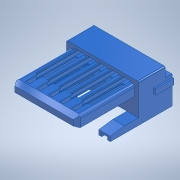
# Autodesk Inventor part: USB 3.0 A Recepticle Insert Fit
Saved by Autodesk Inventor 2020.1 (Build 241239000, 239)
## iProperties
Created: 2019-11-21
Part Number: USB 3.0 A Recepticle Insert Fit
Material: PBT Plastic
Document SubType Name: Modeling
Designer: S. Lee
Mass: 0.400509 g
Surface Area: 10.671 cm^2
Volume: 0.305732 cm^3
Density: 1.31 g/cm^3
Appearance: PBT Blue Pantone 300C
Author: S. Lee
Autodesk Inventor part; units mm, degrees
(part 1 of 2)
ref_plane "YZ Plane" through (0, 0, 0) normal (1, 0, 0) x (0, 1, 0)
ref_plane "XZ Plane" through (0, 0, 0) normal (0, 1, 0) x (-1, 0, 0)
sketch "Sketch1" plane through (0, 0, 0) normal (0, 1, 0) x (-1, 0, 0)
  line L0 (6.55, -2.62) -> (6.55, -5.82)
  line L1 (-6.55, -5.82) -> (-6.55, -2.62)
  line L2 (6.25, -2.62) -> (6.25, 0)
  line L3 (-6.25, 0) -> (-6.25, -2.62)
  line L4 (5.55, 0) -> (5.55, 9.284)
  line L5 (5.05, 10.15) -> (-5.05, 10.15)
  line L6 (-5.55, 9.284) -> (-5.55, 0)
  line L7 (6.25, 0) -> (5.55, 0)
  line L8 (-5.55, 0) -> (-6.25, 0)
  line L9 (-6.55, -2.62) -> (-6.25, -2.62)
  line L10 (6.25, -2.62) -> (6.55, -2.62)
  line L11 (4.605, 9.55) -> (3.395, 9.55)
  line L12 (3.395, 9.55) -> (3.395, 8)
  line L13 (3.395, 8) -> (4.605, 8)
  line L14 (4.605, 8) -> (4.605, 9.55)
  line L15 (2.605, 9.55) -> (1.395, 9.55)
  line L16 (1.395, 9.55) -> (1.395, 8)
  line L17 (1.395, 8) -> (2.605, 8)
  line L18 (2.605, 8) -> (2.605, 9.55)
  line L19 (0.605, 9.55) -> (-0.605, 9.55)
  line L20 (-0.605, 9.55) -> (-0.605, 8)
  line L21 (-0.605, 8) -> (0.605, 8)
  line L22 (0.605, 8) -> (0.605, 9.55)
  line L23 (-1.395, 9.55) -> (-2.605, 9.55)
  line L24 (-2.605, 9.55) -> (-2.605, 8)
  line L25 (-2.605, 8) -> (-1.395, 8)
  line L26 (-1.395, 8) -> (-1.395, 9.55)
  line L27 (-3.395, 9.55) -> (-4.605, 9.55)
  line L28 (-4.605, 9.55) -> (-4.605, 8)
  line L29 (-4.605, 8) -> (-3.395, 8)
  line L30 (-3.395, 8) -> (-3.395, 9.55)
  line L31 (4.05, 6.4) -> (2.95, 6.4)
  line L32 (2.95, 6.4) -> (2.95, -2.82)
  line L33 (4.05, -2.82) -> (4.05, 6.4)
  line L34 (1.55, 6.4) -> (0.45, 6.4)
  line L35 (0.45, 6.4) -> (0.45, -2.82)
  line L36 (1.55, -2.82) -> (1.55, 6.4)
  line L37 (-0.45, 6.4) -> (-1.55, 6.4)
  line L38 (-1.55, 6.4) -> (-1.55, -2.82)
  line L39 (-0.45, -2.82) -> (-0.45, 6.4)
  line L40 (-2.95, 6.4) -> (-4.05, 6.4)
  line L41 (-4.05, 6.4) -> (-4.05, -2.82)
  line L42 (-2.95, -2.82) -> (-2.95, 6.4)
  line L43 (-5.2, -5.82) -> (-5.2, -2.82)
  line L44 (5.2, -2.82) -> (5.2, -5.82)
  line L45 (-5.2, -2.82) -> (-4.05, -2.82)
  line L46 (-2.95, -2.82) -> (-1.55, -2.82)
  line L47 (-0.45, -2.82) -> (0.45, -2.82)
  line L48 (1.55, -2.82) -> (2.95, -2.82)
  line L49 (4.05, -2.82) -> (5.2, -2.82)
  line L50 (6.55, -5.82) -> (5.2, -5.82)
  line L51 (-5.2, -5.82) -> (-6.55, -5.82)
  line L52 (0, -9.014) -> (0, 13.344) projected
  line L53 (4.05, -2.82) -> (2.95, -2.82) construction
  line L54 (1.55, -2.82) -> (0.45, -2.82) construction
  line L55 (-0.45, -2.82) -> (-1.55, -2.82) construction
  line L56 (-2.95, -2.82) -> (-4.05, -2.82) construction
  line L57 (-3.5, 6.4) -> (-3.5, -2.82) construction
  line L58 (-1, 6.4) -> (-1, -2.82) construction
  line L59 (1, 6.4) -> (1, -2.82) construction
  line L60 (3.5, 6.4) -> (3.5, -2.82) construction
  line L61 (5.05, 10.15) -> (5.55, 9.284)
  line L62 (-5.05, 10.15) -> (-5.55, 9.284)
  line L63 (4, 9.55) -> (4, 8) construction
  line L64 (4.605, 8.775) -> (3.395, 8.775) construction
  line L65 (2.605, 8.775) -> (1.395, 8.775) construction
  line L66 (2, 9.55) -> (2, 8) construction
  line L67 (0, 9.55) -> (0, 8) construction
  line L68 (0.605, 8.775) -> (-0.605, 8.775) construction
  line L69 (-1.395, 8.775) -> (-2.605, 8.775) construction
  line L70 (-2, 9.55) -> (-2, 8) construction
  line L71 (-4, 9.55) -> (-4, 8) construction
  line L72 (-3.395, 8.775) -> (-4.605, 8.775) construction
  line L73 (9.17, 0) -> (-9.17, 0) construction
  line L74 (5.55, 5.65) -> (-5.55, 5.65) construction
  point P0 (0, 0)
  point P1 (5.55, 10.15)
  point P2 (-5.55, 10.15)
  dimension "d0" = 10.4
  dimension "d2" = 13.1
  dimension "d3" = 12.5
  dimension "d4" = 11.1
  dimension "d5" = 3.2
  dimension "d6" = 3
  dimension "d7" = 1.1
  dimension "d8" = 1
  dimension "d9" = 1
  dimension "d10" = 3.5
  dimension "d11" = 3.5
  dimension "d12" = 2.15
  dimension "d14" = 1.21
  dimension "d15" = 10.15
  dimension "d16" = 15.97
  dimension "d17" = 0.5
  dimension "d18" = 60
  dimension "d19" = 0.5
  dimension "d20" = 60
  dimension "d21" = 2
  dimension "d22" = 4
  dimension "d23" = 2
  dimension "d24" = 4
  dimension "d25" = 0.6
  dimension "d27" = 4.5
  dimension "d28" = 0.75
  constraints: 146 end point, 30 collinear, 28 midpoint, 22 parallel, 12 horizontal, 12 perpendicular, 6 point on line, 4 other
  measures "d0" distance between parallel lines of L43 L44
  measures "d2" distance between parallel lines of L1 L0
  measures "d3" distance between parallel lines of L3 L2
  measures "d4" distance between parallel lines of L6 L4
  measures "d5" distance of L0.start L0.end
  measures "d6" distance of L44.start L44.end
  measures "d7" distance of L40.start L40.end
  measures "d8" distance between parallel lines of L58 L52
  measures "d9" distance between parallel lines of L52 L59
  measures "d10" distance between parallel lines of L52 L60
  measures "d11" distance between parallel lines of L52 L57
  measures "d12" distance between parallel lines of L5 L29
  measures "d14" distance between parallel lines of L30 L28
  measures "d15" distance of L4.start point (5.55, 10.15)
  measures "d16" distance between parallel lines of L51 L5
  measures "d17" distance of L5.start point (5.55, 10.15)
  measures "d18" angle of L5 L61
  measures "d19" distance of L5.end point (-5.55, 10.15)
  measures "d20" angle of L5 L62
  measures "d21" distance between parallel lines of L66 L52
  measures "d22" distance between parallel lines of L63 L52
  measures "d23" distance between parallel lines of L70 L52
  measures "d24" distance between parallel lines of L71 L52
  measures "d25" distance between parallel lines of L27 L5
  measures "d27" distance between parallel lines of L74 L5
  measures "d28" distance between parallel lines of L74 L40
extrude "Extrusion1" add sketch "Sketch1" along normal blind 0.32 contours L0 L50 L44 L49 L33 L31 L32 L48 L36 L34 L35 L47 L52 L21 L22 L19 L5 L61 L4 L7 L2 L10 | L52 L19 L20 L21 L47 L39 L37 L38 L46 L42 L40 L41 L45 L43 L51 L1 L9 L3 L8 L6 L62 L5
sketch "Sketch2" plane through (0, 0.32, 0) normal (0, 1, 0) x (1, 0, 0)
  line L0 (-4.75, -7.72) -> (4.75, -7.72)
  line L1 (5.55, -9.284) -> (5.55, 0) projected
  line L2 (-5.55, 0) -> (-5.55, -9.284) projected
  line L3 (5.55, -9.284) -> (5.55, 0) projected
  line L4 (5.55, -9.284) -> (5.55, 0)
  line L5 (6.25, 0) -> (6.25, 2.62) projected
  line L6 (6.25, 0) -> (5.55, 0)
  line L7 (6.25, 0) -> (6.25, 5.82)
  line L8 (6.55, 5.82) -> (5.2, 5.82) projected
  line L9 (5.05, -10.15) -> (5.55, -9.284) projected
  line L10 (5.55, -9.284) -> (5.05, -10.15)
  line L11 (5.05, -10.15) -> (-5.05, -10.15)
  line L12 (-5.55, -9.284) -> (-5.05, -10.15) projected
  line L13 (-5.05, -10.15) -> (-5.55, -9.284)
  line L14 (-6.25, 0) -> (-5.55, 0) projected
  line L15 (-5.55, -9.284) -> (-5.55, 0)
  line L16 (-5.55, 0) -> (-6.25, 0)
  line L17 (-6.25, 0) -> (-6.25, 5.82)
  line L18 (-5.2, 5.82) -> (-6.55, 5.82) projected
  line L19 (-5.2, 2.82) -> (-5.2, 5.82) projected
  line L20 (-5.2, 2.82) -> (-5.2, 5.82)
  line L21 (4.75, 2.82) -> (5.2, 2.82)
  line L22 (5.2, 2.82) -> (5.2, 5.82)
  line L23 (-6.25, 5.82) -> (-5.2, 5.82)
  line L24 (5.2, 5.82) -> (6.25, 5.82)
  line L25 (4.75, -7.72) -> (4.75, 2.82)
  line L26 (5.2, 5.82) -> (5.2, 2.82) projected
  line L27 (-4.05, 2.82) -> (-5.2, 2.82) projected
  line L28 (-5.2, 2.82) -> (-4.75, 2.82)
  line L29 (-4.05, 2.82) -> (-5.2, 2.82) projected
  line L30 (-4.75, 2.82) -> (-4.75, -7.72)
  line L31 (5.2, 2.82) -> (4.05, 2.82) projected
  line L32 (-4.605, -8) -> (-3.395, -8) projected
  line L33 (-3.395, -9.55) -> (-4.605, -9.55) projected
  line L34 (-4.605, -9.55) -> (-3.395, -9.55)
  line L35 (-3.395, -9.55) -> (-3.395, -8)
  line L36 (-3.395, -8) -> (-4.605, -8)
  line L37 (-4.605, -8) -> (-4.605, -9.55)
  line L38 (-1.395, -9.55) -> (-2.605, -9.55) projected
  line L39 (-2.605, -8) -> (-1.395, -8) projected
  line L40 (-2.605, -9.55) -> (-1.395, -9.55)
  line L41 (-1.395, -9.55) -> (-1.395, -8)
  line L42 (-1.395, -8) -> (-2.605, -8)
  line L43 (-2.605, -8) -> (-2.605, -9.55)
  line L44 (0.605, -9.55) -> (-0.605, -9.55) projected
  line L45 (0.605, -8) -> (0.605, -9.55) projected
  line L46 (-0.605, -9.55) -> (0.605, -9.55)
  line L47 (0.605, -9.55) -> (0.605, -8)
  line L48 (0.605, -8) -> (-0.605, -8)
  line L49 (-0.605, -8) -> (-0.605, -9.55)
  line L50 (1.395, -9.55) -> (1.395, -8) projected
  line L51 (1.395, -9.55) -> (2.605, -9.55)
  line L52 (2.605, -9.55) -> (2.605, -8)
  line L53 (2.605, -8) -> (1.395, -8)
  line L54 (1.395, -8) -> (1.395, -9.55)
  line L55 (3.395, -9.55) -> (3.395, -8) projected
  line L56 (3.395, -8) -> (4.605, -8) projected
  line L57 (3.395, -9.55) -> (4.605, -9.55)
  line L58 (4.605, -9.55) -> (4.605, -8)
  line L59 (4.605, -8) -> (3.395, -8)
  line L60 (3.395, -8) -> (3.395, -9.55)
  point P0 (0, 0)
  dimension "d34" = 0.8
  dimension "d35" = 0.8
  dimension "d36" = 0.28
  constraints: 76 end point, 12 parallel, 10 perpendicular, 9 horizontal, 8 collinear, 4 point on line, 1 vertical
  measures "d34" distance between parallel lines of L2 L30
  measures "d35" distance between parallel lines of L1 L25
  measures "d36" distance between parallel lines of L0 L32
extrude "Extrusion2" add sketch "Sketch2" along normal blind 0.5
sketch "Sketch3" plane through (0, 0.82, 0) normal (0, 1, 0) x (1, 0, 0)
  line L0 (6.25, 5.82) -> (6.25, 2.62) projected
  line L1 (6.25, 0) -> (6.25, 4.62)
  line L2 (6.25, 4.62) -> (-6.25, 4.62)
  line L3 (-6.25, 4.62) -> (-6.25, 0)
  line L4 (-5.2, 5.82) -> (-6.25, 5.82) projected
  line L5 (-5.55, 0) -> (-5.55, -9.284) projected
  line L6 (-5.55, 0) -> (-5.55, -9.284)
  line L7 (-5.55, -9.284) -> (-5.05, -10.15) projected
  line L8 (-5.55, -9.284) -> (-5.05, -10.15)
  line L9 (5.05, -10.15) -> (5.55, -9.284) projected
  line L10 (-5.05, -10.15) -> (5.05, -10.15)
  line L11 (5.05, -10.15) -> (5.55, -9.284)
  line L12 (5.55, -9.284) -> (5.55, 0) projected
  line L13 (5.55, -9.284) -> (5.55, 0)
  line L14 (-6.25, 0) -> (-5.55, 0)
  line L15 (5.55, 0) -> (6.25, 0)
  line L16 (-5.55, 0) -> (-4.05, 0)
  line L17 (4.05, 0) -> (5.55, 0)
  line L18 (-3.395, -9.55) -> (-4.605, -9.55) projected
  line L19 (-3.395, -8) -> (-3.395, -9.55) projected
  line L20 (-4.605, -9.55) -> (-3.395, -9.55)
  line L21 (-3.395, -9.55) -> (-3.395, -8)
  line L22 (-3.395, -8) -> (-4.605, -8)
  line L23 (-4.605, -8) -> (-4.605, -9.55)
  line L24 (-1.395, -9.55) -> (-2.605, -9.55) projected
  line L25 (-2.605, -8) -> (-1.395, -8) projected
  line L26 (-2.605, -9.55) -> (-1.395, -9.55)
  line L27 (-1.395, -9.55) -> (-1.395, -8)
  line L28 (-1.395, -8) -> (-2.605, -8)
  line L29 (-2.605, -8) -> (-2.605, -9.55)
  line L30 (0.605, -8) -> (0.605, -9.55) projected
  line L31 (-0.605, -9.55) -> (0.605, -9.55)
  line L32 (0.605, -9.55) -> (0.605, -8)
  line L33 (0.605, -8) -> (-0.605, -8)
  line L34 (-0.605, -8) -> (-0.605, -9.55)
  line L35 (2.605, -9.55) -> (1.395, -9.55) projected
  line L36 (1.395, -9.55) -> (2.605, -9.55)
  line L37 (2.605, -9.55) -> (2.605, -8)
  line L38 (2.605, -8) -> (1.395, -8)
  line L39 (1.395, -8) -> (1.395, -9.55)
  line L40 (4.605, -9.55) -> (3.395, -9.55) projected
  line L41 (3.395, -8) -> (4.605, -8) projected
  line L42 (3.395, -9.55) -> (4.605, -9.55)
  line L43 (4.605, -9.55) -> (4.605, -8)
  line L44 (4.605, -8) -> (3.395, -8)
  line L45 (3.395, -8) -> (3.395, -9.55)
  line L46 (5.55, 0) -> (6.25, 0) projected
  line L47 (-6.25, 4.62) -> (6.25, 4.62)
  line L48 (6.25, 4.62) -> (6.25, 0)
  line L49 (6.25, 0) -> (-6.25, 0)
  line L50 (-6.25, 0) -> (-6.25, 4.62)
  line L51 (-4.605, -7.4) -> (-3.395, -7.4)
  line L52 (-3.395, -7.4) -> (-3.395, 0)
  line L53 (-3.395, 0) -> (-4.605, 0)
  line L54 (-4.605, 0) -> (-4.605, -7.4)
  line L55 (-2.605, -7.4) -> (-1.395, -7.4)
  line L56 (-1.395, -7.4) -> (-1.395, 0)
  line L57 (-1.395, 0) -> (-2.605, 0)
  line L58 (-2.605, 0) -> (-2.605, -7.4)
  line L59 (-0.605, -7.4) -> (0.605, -7.4)
  line L60 (0.605, -7.4) -> (0.605, 0)
  line L61 (0.605, 0) -> (-0.605, 0)
  line L62 (-0.605, 0) -> (-0.605, -7.4)
  line L63 (1.395, -7.4) -> (2.605, -7.4)
  line L64 (2.605, -7.4) -> (2.605, 0)
  line L65 (2.605, 0) -> (1.395, 0)
  line L66 (1.395, 0) -> (1.395, -7.4)
  line L67 (3.395, 0) -> (4.605, 0)
  line L68 (4.605, 0) -> (4.605, -7.4)
  line L69 (4.605, -7.4) -> (3.395, -7.4)
  line L70 (3.395, -7.4) -> (3.395, 0)
  line L71 (-4.605, -9.55) -> (-4.605, -8) projected
  line L72 (-3.395, -8) -> (-3.395, -9.55) projected
  line L73 (-2.605, -9.55) -> (-2.605, -8) projected
  line L74 (-1.395, -8) -> (-1.395, -9.55) projected
  line L75 (-0.605, -9.55) -> (-0.605, -8) projected
  line L76 (0.605, -8) -> (0.605, -9.55) projected
  line L77 (1.395, -9.55) -> (1.395, -8) projected
  line L78 (2.605, -8) -> (2.605, -9.55) projected
  line L79 (3.395, -9.55) -> (3.395, -8) projected
  line L80 (4.605, -8) -> (4.605, -9.55) projected
  point P0 (-0.605, 0)
  dimension "d39" = 1.2
  dimension "d88" = 0.6
  constraints: 112 end point, 25 parallel, 17 collinear, 14 perpendicular, 10 horizontal, 6 point on line, 1 vertical
  measures "d39" distance between parallel lines of L2 L4
  measures "d88" distance between parallel lines of L51 L22
extrude "Extrusion3" add sketch "Sketch3" along normal blind 0.02 contours L0 L1 L15 L17 L49 L16 L14 L3 L2 | L12 L9 L10 L7 L5 L16 L54 L51 L52 L49 L58 L55 L56 L62 L59 L60 L66 L63 L64 L70 L69 L68 L17
sketch "Sketch5" plane through (0, 0.84, 0) normal (0, 1, 0) x (1, 0, 0)
  line L0 (-6.25, 0) -> (-5.55, 0) projected
  line L1 (5.2, 4.62) -> (6.25, 4.62) projected
  line L2 (-6.25, 0) -> (6.25, 0)
  line L3 (6.25, 0) -> (6.25, 4.62)
  line L4 (6.25, 4.62) -> (-6.25, 4.62)
  line L5 (-6.25, 4.62) -> (-6.25, 0)
  line L6 (-4.605, 0) -> (-3.395, 0) projected
  line L7 (-3.395, -8) -> (-3.395, -9.55) projected
  line L8 (-4.605, 0) -> (-3.395, 0)
  line L9 (-3.395, 0) -> (-3.395, -9.05)
  line L10 (-3.395, -9.05) -> (-4.605, -9.05)
  line L11 (-4.605, -9.05) -> (-4.605, 0)
  line L12 (-2.605, -7.4) -> (-2.605, 0) projected
  line L13 (-1.395, -8) -> (-1.395, -9.55) projected
  line L14 (-2.605, 0) -> (-1.395, 0)
  line L15 (-1.395, 0) -> (-1.395, -9.05)
  line L16 (-1.395, -9.05) -> (-2.605, -9.05)
  line L17 (-2.605, -9.05) -> (-2.605, 0)
  line L18 (-0.605, 0) -> (0.605, 0) projected
  line L19 (0.605, -8) -> (0.605, -9.55) projected
  line L20 (-0.605, 0) -> (0.605, 0)
  line L21 (0.605, 0) -> (0.605, -9.05)
  line L22 (0.605, -9.05) -> (-0.605, -9.05)
  line L23 (-0.605, -9.05) -> (-0.605, 0)
  line L24 (1.395, 0) -> (2.605, 0) projected
  line L25 (2.605, -8) -> (2.605, -9.55) projected
  line L26 (1.395, 0) -> (2.605, 0)
  line L27 (2.605, 0) -> (2.605, -9.05)
  line L28 (2.605, -9.05) -> (1.395, -9.05)
  line L29 (1.395, -9.05) -> (1.395, 0)
  line L30 (3.395, 0) -> (4.605, 0) projected
  line L31 (4.605, -8) -> (4.605, -9.55) projected
  line L32 (3.395, 0) -> (4.605, 0)
  line L33 (4.605, 0) -> (4.605, -9.05)
  line L34 (4.605, -9.05) -> (3.395, -9.05)
  line L35 (3.395, -9.05) -> (3.395, 0)
  line L36 (-3.395, -9.55) -> (-4.605, -9.55) projected
  line L37 (-5.55, 0) -> (-5.55, -9.284) projected
  line L38 (-5.55, 0) -> (-5.55, -9.284)
  line L39 (-5.55, -9.284) -> (-5.05, -10.15)
  line L40 (-5.05, -10.15) -> (5.05, -10.15) projected
  line L41 (-5.05, -10.15) -> (5.05, -10.15)
  line L42 (5.05, -10.15) -> (5.55, -9.284) projected
  line L43 (5.05, -10.15) -> (5.55, -9.284)
  line L44 (5.55, 0) -> (6.25, 0) projected
  line L45 (5.55, -9.284) -> (5.55, 0)
  point P0 (-2.605, -7.4)
  dimension "d93" = 0.5
  constraints: 56 end point, 11 parallel, 9 point on line, 6 horizontal, 6 perpendicular, 3 collinear, 1 vertical, 3 other
  measures "d93" distance between parallel lines of L10 L36
extrude "Extrusion5" add sketch "Sketch5" along normal blind 0.09 contours L5 L4 L1 L3 L2 L0 | L2 L11 L10 L7 L9 L12 L17 L16 L13 L15 L23 L22 L19 L21 L29 L28 L25 L27 L35 L34 L31 L33 L45 L42 L40 L39 L37
sketch "Sketch6" plane through (0, 0.93, 0) normal (0, 1, 0) x (1, 0, 0)
  line L0 (-4.605, -9.05) -> (-4.605, 0) projected
  line L1 (-3.395, 0) -> (-3.395, -9.05) projected
  line L2 (-4.605, -9.05) -> (-3.395, -9.05)
  line L3 (-3.395, -9.05) -> (-3.395, -6.9)
  line L4 (-3.395, -6.9) -> (-4.605, -6.9)
  line L5 (-4.605, -6.9) -> (-4.605, -9.05)
  line L6 (-3.395, -7.4) -> (-4.605, -7.4) projected
  line L7 (-2.605, -9.05) -> (-2.605, 0) projected
  line L8 (-1.395, 0) -> (-1.395, -7.4) projected
  line L9 (-2.605, -9.05) -> (-1.395, -9.05)
  line L10 (-1.395, -9.05) -> (-1.395, -6.9)
  line L11 (-1.395, -6.9) -> (-2.605, -6.9)
  line L12 (-2.605, -6.9) -> (-2.605, -9.05)
  line L13 (-0.605, -9.05) -> (-0.605, 0) projected
  line L14 (0.605, 0) -> (0.605, -9.05) projected
  line L15 (-0.605, -9.05) -> (0.605, -9.05)
  line L16 (0.605, -9.05) -> (0.605, -6.9)
  line L17 (0.605, -6.9) -> (-0.605, -6.9)
  line L18 (-0.605, -6.9) -> (-0.605, -9.05)
  line L19 (1.395, -9.55) -> (1.395, -8) projected
  line L20 (2.605, 0) -> (2.605, -7.4) projected
  line L21 (1.395, -9.05) -> (2.605, -9.05)
  line L22 (2.605, -9.05) -> (2.605, -6.9)
  line L23 (2.605, -6.9) -> (1.395, -6.9)
  line L24 (1.395, -6.9) -> (1.395, -9.05)
  line L25 (3.395, -9.55) -> (3.395, -8) projected
  line L26 (3.395, -9.05) -> (4.605, -9.05)
  line L27 (4.605, -9.05) -> (4.605, -6.9)
  line L28 (4.605, -6.9) -> (3.395, -6.9)
  line L29 (3.395, -6.9) -> (3.395, -9.05)
  line L30 (-4.75, -6.9) -> (-3.25, -6.9)
  line L31 (-3.25, -6.9) -> (-3.25, 4.62)
  line L32 (-3.25, 4.62) -> (-4.75, 4.62)
  line L33 (-4.75, 4.62) -> (-4.75, -6.9)
  line L34 (6.25, 4.62) -> (-6.25, 4.62) projected
  line L35 (5.2, 4.62) -> (-5.2, 4.62) projected
  line L36 (-2.75, -6.9) -> (-1.25, -6.9)
  line L37 (-1.25, -6.9) -> (-1.25, 4.62)
  line L38 (-1.25, 4.62) -> (-2.75, 4.62)
  line L39 (-2.75, 4.62) -> (-2.75, -6.9)
  line L40 (-0.75, -6.9) -> (0.75, -6.9)
  line L41 (0.75, -6.9) -> (0.75, 4.62)
  line L42 (0.75, 4.62) -> (-0.75, 4.62)
  line L43 (-0.75, 4.62) -> (-0.75, -6.9)
  line L44 (1.25, -6.9) -> (2.75, -6.9)
  line L45 (2.75, -6.9) -> (2.75, 4.62)
  line L46 (2.75, 4.62) -> (1.25, 4.62)
  line L47 (1.25, 4.62) -> (1.25, -6.9)
  line L48 (3.25, -6.9) -> (4.75, -6.9)
  line L49 (4.75, -6.9) -> (4.75, 4.62)
  line L50 (4.75, 4.62) -> (3.25, 4.62)
  line L51 (3.25, 4.62) -> (3.25, -6.9)
  line L52 (4.605, 0) -> (4.605, -9.05) projected
  line L53 (-6.25, 4.62) -> (-5.2, 4.62) projected
  line L54 (5.55, 0) -> (6.25, 0) projected
  line L55 (-6.25, 4.62) -> (6.25, 4.62)
  line L56 (6.25, 4.62) -> (6.25, 0)
  line L57 (6.25, 0) -> (-6.25, 0)
  line L58 (-6.25, 0) -> (-6.25, 4.62)
  line L59 (-5.55, 0) -> (-5.55, -9.284) projected
  line L60 (-5.55, -9.284) -> (-5.05, -10.15) projected
  line L61 (-5.55, 0) -> (-5.55, -9.284)
  line L62 (-5.55, -9.284) -> (-5.05, -10.15) projected
  line L63 (-5.55, -9.284) -> (-5.05, -10.15)
  line L64 (-5.05, -10.15) -> (5.05, -10.15)
  line L65 (5.05, -10.15) -> (5.55, -9.284) projected
  line L66 (5.05, -10.15) -> (5.55, -9.284)
  line L67 (5.55, -9.284) -> (5.55, 0) projected
  line L68 (5.55, -9.284) -> (5.55, 0)
  point P0 (0, 0)
  point P1 (-0.75, 4.62)
  point P2 (-3.25, 4.62)
  dimension "d94" = 0.5
  dimension "d95" = 1.5
  dimension "d96" = 0.145
  dimension "d97" = 0.145
  dimension "d99" = 1.5
  dimension "d100" = 1.5
  dimension "d101" = 1.5
  dimension "d102" = 1.5
  dimension "d103" = 0.145
  dimension "d104" = 0.145
  dimension "d105" = 0.145
  dimension "d106" = 0.145
  dimension "d107" = 0.145
  dimension "d108" = 0.145
  dimension "d109" = 0.145
  dimension "d110" = 0.145
  constraints: 98 end point, 25 equal length, 18 point on line, 12 perpendicular, 11 horizontal, 5 collinear, 1 vertical
  measures "d94" distance between parallel lines of L6 L4
  measures "d95" distance between parallel lines of L31 L33
  measures "d96" distance between parallel lines of L5 L33
  measures "d97" distance between parallel lines of L1 L31
  measures "d99" distance between parallel lines of L37 L39
  measures "d100" distance between parallel lines of L41 L43
  measures "d101" distance between parallel lines of L45 L47
  measures "d102" distance between parallel lines of L49 L51
  measures "d103" distance between parallel lines of L7 L39
  measures "d104" distance between parallel lines of L37 L8
  measures "d105" distance between parallel lines of L13 L43
  measures "d106" distance between parallel lines of L16 L41
  measures "d107" distance between parallel lines of L47 L24
  measures "d108" distance between parallel lines of L45 L22
  measures "d109" distance between parallel lines of L29 L51
  measures "d110" distance between parallel lines of L49 L52
extrude "Extrusion6" add sketch "Sketch6" along normal blind 0.55 contours L2 L1 L30 L31 L57 L39 L36 L7 L9 L10 L8 L37 L43 L40 L13 L15 L14 L41 L47 L44 L24 L19 L21 L22 L20 L45 L51 L48 L29 L25 L26 L27 L49 L67 L65 L64 L60 L59 L33 L0 | L57 L58 L34 L33 | L31 L34 L39 L57 | L34 L43 L57 L37 | L34 L47 L57 L41 | L57 L49 L34 L56 L54 | L34 L51 L57 L45
sketch "Sketch7" plane through (0, 1.48, 0) normal (0, 1, 0) x (1, 0, 0)
  line L0 (5.2, 4.62) -> (-5.2, 4.62) projected
  line L1 (-4.8, 4.62) -> (-3.2, 4.62)
  line L2 (-3.2, 4.62) -> (-3.2, -6.9)
  line L3 (-3.2, -6.9) -> (-4.8, -6.9)
  line L4 (-4.8, -6.9) -> (-4.8, 4.62)
  line L5 (-4.75, -6.9) -> (-4.75, 4.62) projected
  line L6 (-3.25, 4.62) -> (-3.25, -6.9) projected
  line L7 (-4.605, -6.9) -> (-4.75, -6.9) projected
  line L8 (-3.395, -9.05) -> (-4.605, -9.05) projected
  line L9 (-3.25, -6.9) -> (-3.395, -6.9) projected
  line L10 (-4.605, -9.05) -> (-3.395, -9.05)
  line L11 (-3.395, -9.05) -> (-3.395, -6.9)
  line L12 (-3.395, -6.9) -> (-4.605, -6.9)
  line L13 (-4.605, -6.9) -> (-4.605, -9.05)
  line L14 (-1.2, 4.62) -> (-1.2, -6.9)
  line L15 (-2.8, -6.9) -> (-2.8, 4.62)
  line L16 (-2.8, 4.62) -> (-1.2, 4.62)
  line L17 (-1.2, -6.9) -> (-2.8, -6.9)
  line L18 (-1.395, -6.9) -> (-2.605, -6.9)
  line L19 (-2.605, -9.05) -> (-1.395, -9.05)
  line L20 (-1.395, -9.05) -> (-1.395, -6.9)
  line L21 (-2.605, -6.9) -> (-2.605, -9.05)
  line L22 (0.8, 4.62) -> (0.8, -6.9)
  line L23 (-0.8, -6.9) -> (-0.8, 4.62)
  line L24 (-0.8, 4.62) -> (0.8, 4.62)
  line L25 (0.8, -6.9) -> (-0.8, -6.9)
  line L26 (0.605, -6.9) -> (-0.605, -6.9)
  line L27 (-0.605, -9.05) -> (0.605, -9.05)
  line L28 (0.605, -9.05) -> (0.605, -6.9)
  line L29 (-0.605, -6.9) -> (-0.605, -9.05)
  line L30 (2.8, 4.62) -> (2.8, -6.9)
  line L31 (1.2, -6.9) -> (1.2, 4.62)
  line L32 (1.2, 4.62) -> (2.8, 4.62)
  line L33 (2.8, -6.9) -> (1.2, -6.9)
  line L34 (2.605, -6.9) -> (1.395, -6.9)
  line L35 (1.395, -9.05) -> (2.605, -9.05)
  line L36 (2.605, -9.05) -> (2.605, -6.9)
  line L37 (1.395, -6.9) -> (1.395, -9.05)
  line L38 (4.8, 4.62) -> (4.8, -6.9)
  line L39 (3.2, -6.9) -> (3.2, 4.62)
  line L40 (3.2, 4.62) -> (4.8, 4.62)
  line L41 (4.8, -6.9) -> (3.2, -6.9)
  line L42 (4.605, -6.9) -> (3.395, -6.9)
  line L43 (3.395, -9.05) -> (4.605, -9.05)
  line L44 (4.605, -9.05) -> (4.605, -6.9)
  line L45 (3.395, -6.9) -> (3.395, -9.05)
  line L46 (-6.25, 4.62) -> (-5.2, 4.62) projected
  line L47 (-4.8, 4.62) -> (-6.25, 4.62)
  line L48 (-6.25, 2.62) -> (-6.25, 0) projected
  line L49 (-6.25, 4.62) -> (-6.25, 0)
  line L50 (-6.25, 0) -> (-5.55, 0) projected
  line L51 (-6.25, 0) -> (-5.55, 0)
  line L52 (-5.55, 0) -> (-5.55, -9.284) projected
  line L53 (-5.55, 0) -> (-5.55, -9.284)
  line L54 (-5.55, -9.284) -> (-5.05, -10.15) projected
  line L55 (-5.55, -9.284) -> (-5.05, -10.15)
  line L56 (-5.05, -10.15) -> (5.05, -10.15)
  line L57 (5.05, -10.15) -> (5.55, -9.284) projected
  line L58 (5.05, -10.15) -> (5.55, -9.284)
  line L59 (5.55, -9.284) -> (5.55, 0) projected
  line L60 (5.55, -9.284) -> (5.55, 0)
  line L61 (5.55, 0) -> (6.25, 0) projected
  line L62 (5.55, 0) -> (6.25, 0)
  line L63 (6.25, 4.62) -> (6.25, 5.82) projected
  line L64 (6.25, 0) -> (6.25, 4.62)
  line L65 (6.25, 4.62) -> (4.75, 4.62) projected
  line L66 (6.25, 4.62) -> (4.75, 4.62)
  line L67 (2.8, 4.62) -> (3.2, 4.62)
  line L68 (3.25, 4.62) -> (2.75, 4.62) projected
  line L69 (0.8, 4.62) -> (1.2, 4.62)
  line L70 (-1.2, 4.62) -> (-0.8, 4.62)
  line L71 (-3.2, 4.62) -> (-2.8, 4.62)
  point P0 (0, 0)
  point P1 (-2.75, -6.9)
  point P2 (-1.25, -6.9)
  point P3 (-0.75, -6.9)
  point P4 (0.75, -6.9)
  point P5 (1.25, -6.9)
  point P6 (2.75, -6.9)
  point P7 (3.25, -6.9)
  point P8 (4.75, -6.9)
  point P9 (3.2, 4.62)
  point P10 (-2.8, 4.62)
  point P11 (-4.605, -6.9)
  dimension "d113" = 0.05
  dimension "d114" = 0.05
  dimension "d117" = 2
  constraints: 110 end point, 13 collinear, 5 parallel, 4 perpendicular, 3 horizontal, 1 point on line, 72 other
  measures "d113" distance between parallel lines of L4 L5
  measures "d114" distance between parallel lines of L6 L2
  measures "d117" distance of L1.end L14.start
extrude "Extrusion7" add sketch "Sketch7" along normal blind 0.2 contours L65 L64 L61 L59 L57 L56 L54 L52 L50 L48 L49 L46 L0 L4 L3 L13 L8 L11 L2 L15 L17 L21 L19 L20 L14 L23 L25 L29 L27 L28 L22 L31 L33 L37 L35 L36 L30 L39 L41 L45 L43 L44 L38
sketch "Sketch8" plane through (0, 1.68, 0) normal (0, 1, 0) x (1, 0, 0)
  line L0 (-4.355, -9.05) -> (-4.355, -6.9)
  line L1 (-3.645, -6.9) -> (-3.645, -9.05)
  line L2 (-4.355, -9.05) -> (-3.645, -9.05)
  line L3 (-3.645, -9.05) -> (-3.645, -6.9)
  line L4 (-4.355, -6.9) -> (-4.355, -9.05)
  line L5 (-2.355, -9.05) -> (-2.355, -6.9)
  line L6 (-2.355, -9.05) -> (-1.645, -9.05)
  line L7 (-1.645, -9.05) -> (-1.645, -6.9)
  line L8 (-2.355, -6.9) -> (-2.355, -9.05)
  line L9 (-0.355, -9.05) -> (-0.355, -6.9)
  line L10 (0.355, -6.9) -> (0.355, -9.05)
  line L11 (-0.355, -9.05) -> (0.355, -9.05)
  line L12 (0.355, -9.05) -> (0.355, -6.9)
  line L13 (-0.355, -6.9) -> (-0.355, -9.05)
  line L14 (1.645, -9.05) -> (2.355, -9.05)
  line L15 (2.355, -9.05) -> (2.355, -6.9)
  line L16 (1.645, -6.9) -> (1.645, -9.05)
  line L17 (3.645, -9.05) -> (4.355, -9.05)
  line L18 (4.355, -9.05) -> (4.355, -6.9)
  line L19 (3.645, -6.9) -> (3.645, -9.05)
  line L20 (-3.25, -6.9) -> (-3.25, 4.62)
  line L21 (-4.75, 4.62) -> (-4.75, -6.9)
  line L22 (-1.25, -6.9) -> (-1.25, 4.62)
  line L23 (-2.75, 4.62) -> (-2.75, -6.9)
  line L24 (0.75, -6.9) -> (0.75, 4.62)
  line L25 (-0.75, 4.62) -> (-0.75, -6.9)
  line L26 (2.75, -6.9) -> (2.75, 4.62)
  line L27 (1.25, 4.62) -> (1.25, -6.9)
  line L28 (4.75, -6.9) -> (4.75, 4.62)
  line L29 (3.25, 4.62) -> (3.25, -6.9)
  line L30 (4.355, -6.9) -> (4.355, -9.05)
  line L31 (6.25, 4.62) -> (6.25, 0)
  line L32 (-6.25, 0) -> (-6.25, 4.62)
  line L33 (-5.55, 0) -> (-5.55, -9.284)
  line L34 (-5.55, -9.284) -> (-5.05, -10.15)
  line L35 (-5.55, 0) -> (-5.55, -9.284)
  line L36 (-5.55, -9.284) -> (-5.05, -10.15)
  line L37 (-5.55, -9.284) -> (-5.05, -10.15)
  line L38 (-5.05, -10.15) -> (5.05, -10.15)
  line L39 (5.05, -10.15) -> (5.55, -9.284)
  line L40 (5.05, -10.15) -> (5.55, -9.284)
  line L41 (5.55, -9.284) -> (5.55, 0)
  line L42 (5.55, -9.284) -> (5.55, 0)
  line L43 (5.55, -9.284) -> (5.55, 0) projected
  line L44 (5.05, -10.15) -> (5.55, -9.284) projected
  line L45 (-5.05, -10.15) -> (5.05, -10.15) projected
  line L46 (-5.55, -9.284) -> (-5.05, -10.15) projected
  line L47 (-5.55, 0) -> (-5.55, -9.284) projected
  line L48 (-6.25, 0) -> (-5.55, 0) projected
  line L49 (-6.25, 4.62) -> (-6.25, 0) projected
  line L50 (-4.8, 4.62) -> (-6.25, 4.62) projected
  line L51 (-4.75, -6.9) -> (-4.355, -6.9)
  line L52 (-3.645, -6.9) -> (-3.25, -6.9)
  line L53 (-2.75, -6.9) -> (-2.355, -6.9)
  line L54 (-1.645, -6.9) -> (-1.25, -6.9)
  line L55 (-0.75, -6.9) -> (-0.355, -6.9)
  line L56 (0.355, -6.9) -> (0.75, -6.9)
  line L57 (1.25, -6.9) -> (1.645, -6.9)
  line L58 (2.355, -6.9) -> (2.75, -6.9)
  line L59 (3.25, -6.9) -> (3.645, -6.9)
  line L60 (4.355, -6.9) -> (4.75, -6.9)
  line L61 (-4.75, -6.9) -> (-4.75, 4.62) projected
  line L62 (-3.25, 4.62) -> (-3.25, -6.9) projected
  line L63 (-2.75, -6.9) -> (-2.75, 4.62) projected
  line L64 (-1.25, 4.62) -> (-1.25, -6.9) projected
  line L65 (-0.75, -6.9) -> (-0.75, 4.62) projected
  line L66 (0.75, 4.62) -> (0.75, -6.9) projected
  line L67 (1.25, -6.9) -> (1.25, 4.62) projected
  line L68 (2.75, 4.62) -> (2.75, -6.9) projected
  line L69 (3.25, -6.9) -> (3.25, 4.62) projected
  line L70 (4.75, 4.62) -> (4.75, -6.9) projected
  line L71 (-4.605, -6.9) -> (-4.8, -6.9) projected
  line L72 (-3.2, -6.9) -> (-3.395, -6.9) projected
  line L73 (-3.395, -9.05) -> (-4.605, -9.05) projected
  line L74 (-1.395, -9.05) -> (-2.605, -9.05) projected
  line L75 (0.605, -9.05) -> (-0.605, -9.05) projected
  line L76 (6.25, 0) -> (6.25, 4.62) projected
  line L77 (6.25, 0) -> (5.55, 0)
  line L78 (4.75, 0) -> (3.25, 0)
  line L79 (4.75, 4.62) -> (6.25, 4.62)
  line L80 (6.3774, 4.62) -> (4.75, 4.62)
  line L81 (3.25, 4.62) -> (2.75, 4.62)
  line L82 (2.75, 4.62) -> (3.25, 4.62)
  line L83 (2.75, 0) -> (1.25, 0)
  line L84 (1.25, 4.62) -> (0.75, 4.62)
  line L85 (0.75, 4.62) -> (1.25, 4.62)
  line L86 (0.75, 0) -> (-0.75, 0)
  line L87 (-0.75, 4.62) -> (-1.25, 4.62)
  line L88 (-1.25, 4.62) -> (-0.75, 4.62)
  line L89 (-1.25, 0) -> (-2.75, 0)
  line L90 (-2.75, 4.62) -> (-3.25, 4.62)
  line L91 (-4.75, 4.62) -> (-6.25, 4.62)
  line L92 (-6.25, 4.62) -> (-4.75, 4.62)
  line L93 (-3.25, 4.62) -> (-2.75, 4.62)
  line L94 (-3.25, 0) -> (-4.75, 0)
  line L95 (-5.55, 0) -> (-6.25, 0)
  line L96 (-4.605, -9.05) -> (-4.605, -6.9) projected
  line L97 (-3.395, -6.9) -> (-3.395, -9.05) projected
  line L98 (-2.605, -9.05) -> (-2.605, -6.9) projected
  line L99 (-1.395, -6.9) -> (-1.395, -9.05) projected
  line L100 (-0.605, -9.05) -> (-0.605, -6.9) projected
  line L101 (0.605, -6.9) -> (0.605, -9.05) projected
  line L102 (1.395, -9.05) -> (1.395, -6.9) projected
  line L103 (2.605, -6.9) -> (2.605, -9.05) projected
  line L104 (3.395, -9.05) -> (3.395, -6.9) projected
  line L105 (4.605, -6.9) -> (4.605, -9.05) projected
  point P0 (0, 0)
  point P1 (0, 0)
  point P2 (4.605, -6.9)
  point P3 (3.395, -8)
  point P4 (3.395, -6.9)
  point P5 (2.605, -6.9)
  point P6 (2.605, -7.4)
  point P7 (1.395, -8)
  point P8 (1.395, -6.9)
  point P9 (1.25, 4.62)
  point P10 (0.75, 4.62)
  point P11 (0.605, -6.9)
  point P12 (0.605, -9.05)
  point P13 (-0.605, -6.9)
  point P14 (-0.75, 4.62)
  point P15 (-1.395, -6.9)
  point P16 (-1.395, -7.4)
  point P17 (-2.605, -6.9)
  point P18 (-2.75, 4.62)
  point P19 (-4.605, -6.9)
  point P20 (-4.75, 4.62)
  point P21 (-4.8, 4.62)
  dimension "d151" = 0.25
  dimension "d152" = 0.25
  dimension "d153" = 0.25
  dimension "d154" = 0.25
  dimension "d155" = 0.25
  dimension "d156" = 0.25
  dimension "d157" = 0.25
  dimension "d158" = 0.25
  dimension "d159" = 0.25
  dimension "d160" = 0.25
  constraints: 155 end point, 48 parallel, 38 collinear, 22 perpendicular, 21 horizontal, 12 point on line, 1 vertical
  measures "d151" distance between parallel lines of L0 L96
  measures "d152" distance between parallel lines of L97 L1
  measures "d153" distance between parallel lines of L98 L5
  measures "d154" distance between parallel lines of L99 L7
  measures "d155" distance between parallel lines of L100 L9
  measures "d156" distance between parallel lines of L101 L10
  measures "d157" distance between parallel lines of L102 L16
  measures "d158" distance between parallel lines of L103 L15
  measures "d159" distance between parallel lines of L104 L19
  measures "d160" distance between parallel lines of L105 L18
extrude "Extrusion8" add sketch "Sketch8" along normal blind 0.16 contours L73 L96 L51 L0 | L2 L73 L97 L52 L20 L90 L23 L53 L98 L74 L6 L99 L54 L22 L87 L25 L55 L100 L75 L11 L101 L56 L24 L84 L27 L57 L16 L14 L15 L58 L26 L81 L29 L59 L19 L17 L18 L60 L28 L79 L31 L77 L41 L39 L38 L34 L33 L48 L32 L50 L91 L21 L51 L96 | L1 L52 L97 L73 | L53 L5 L74 L98 | L99 L74 L7 L54 | L55 L9 L75 L100 | L101 L75 L10 L56
sketch "Sketch10" plane through (0, 1.84, 0) normal (0, 1, 0) x (1, 0, 0)
  line L0 (-6.25, 4.62) -> (-6.25, 0) projected
  line L1 (-4.75, -6.9) -> (-4.75, 4.62) projected
  line L2 (-6.25, 0) -> (-4.75, 0)
  line L3 (-4.75, 0) -> (-4.75, 4.62)
  line L4 (-4.75, 4.62) -> (-6.25, 4.62)
  line L5 (-6.25, 4.62) -> (-6.25, 0)
  line L6 (-3.25, 4.62) -> (-3.25, -6.9) projected
  line L7 (-2.75, -6.9) -> (-2.75, 4.62) projected
  line L8 (-3.25, 0) -> (-2.75, 0)
  line L9 (-2.75, 0) -> (-2.75, 4.62)
  line L10 (-2.75, 4.62) -> (-3.25, 4.62)
  line L11 (-3.25, 4.62) -> (-3.25, 0)
  line L12 (-1.25, 4.62) -> (-1.25, -6.9) projected
  line L13 (-0.75, -6.9) -> (-0.75, 4.62) projected
  line L14 (-1.25, 0) -> (-0.75, 0)
  line L15 (-0.75, 0) -> (-0.75, 4.62)
  line L16 (-0.75, 4.62) -> (-1.25, 4.62)
  line L17 (-1.25, 4.62) -> (-1.25, 0)
  line L18 (0.75, 4.62) -> (-0.75, 4.62) projected
  line L19 (1.25, 4.62) -> (1.25, -6.9) projected
  line L20 (0.75, 4.62) -> (1.25, 4.62)
  line L21 (1.25, 4.62) -> (1.25, 0)
  line L22 (1.25, 0) -> (0.75, 0)
  line L23 (0.75, 0) -> (0.75, 4.62)
  line L24 (2.75, 4.62) -> (2.75, -6.9) projected
  line L25 (4.75, 4.62) -> (3.25, 4.62) projected
  line L26 (2.75, 0) -> (3.25, 0)
  line L27 (3.25, 0) -> (3.25, 4.62)
  line L28 (3.25, 4.62) -> (2.75, 4.62)
  line L29 (2.75, 4.62) -> (2.75, 0)
  line L30 (4.75, 4.62) -> (4.75, -6.9) projected
  line L31 (6.25, 0) -> (6.25, 4.62) projected
  line L32 (4.75, 4.62) -> (6.25, 4.62)
  line L33 (6.25, 4.62) -> (6.25, 0)
  line L34 (6.25, 0) -> (4.75, 0)
  line L35 (4.75, 0) -> (4.75, 4.62)
  point P0 (6.25, 4.62)
  point P1 (-1.25, 4.62)
  point P2 (-3.25, 4.62)
  point P3 (-6.25, 4.62)
  constraints: 48 end point, 12 parallel, 8 point on line, 6 horizontal, 6 perpendicular
extrude "Extrusion10" add sketch "Sketch10" along normal blind 0.22
sketch "Sketch11" plane through (0, 2.06, 0) normal (0, 1, 0) x (1, 0, 0)
  line L0 (-6.25, 0) -> (-5.55, 0) projected
  line L1 (6.25, 4.62) -> (4.75, 4.62) projected
  line L2 (-6.25, 0) -> (6.25, 0)
  line L3 (6.25, 0) -> (6.25, 4.62)
  line L4 (6.25, 4.62) -> (-6.25, 4.62)
  line L5 (-6.25, 4.62) -> (-6.25, 0)
  point P0 (0, 0)
  constraints: 8 end point, 2 parallel, 1 horizontal, 1 perpendicular
extrude "Extrusion11" add sketch "Sketch11" along normal blind 0.5
sketch "Sketch12" plane through (0, 0, 0) normal (0, -1, 0) x (1, 0, 0)
  line L0 (-4.05, 6.4) -> (-4.05, -2.82) projected
  line L1 (-6.25, -2.62) -> (-6.25, -5.82) projected
  line L2 (-4.05, 0) -> (-6.25, 0)
  line L3 (-6.25, 0) -> (-6.25, -2.62)
  line L4 (-5.2, -2.82) -> (-4.05, -2.82)
  line L5 (-4.05, -2.82) -> (-4.05, 0)
  line L6 (-5.2, -5.82) -> (-6.25, -5.82) projected
  line L7 (-6.55, -5.82) -> (-6.55, -2.62) projected
  line L8 (-5.2, -5.82) -> (-6.55, -5.82)
  line L9 (-6.55, -5.82) -> (-6.55, -2.62)
  line L10 (-6.55, -2.62) -> (-6.25, -2.62)
  line L11 (-5.2, -2.82) -> (-5.2, -5.82)
  line L12 (-4.05, -2.82) -> (-5.2, -2.82) projected
  line L13 (-6.25, 0) -> (-5.55, 0) projected
  line L14 (-6.25, -2.62) -> (-6.25, 0) projected
  line L15 (-1.55, -2.82) -> (-2.95, -2.82) projected
  line L16 (-2.95, -2.82) -> (-2.95, 6.4) projected
  line L17 (-1.55, -2.82) -> (-2.95, -2.82)
  line L18 (-2.95, -2.82) -> (-2.95, 0)
  line L19 (-2.95, 0) -> (-1.55, 0)
  line L20 (-1.55, 0) -> (-1.55, -2.82)
  line L21 (-0.45, -2.82) -> (-0.45, 6.4) projected
  line L22 (0.45, 6.4) -> (0.45, -2.82) projected
  line L23 (-0.45, 0) -> (0.45, 0)
  line L24 (0.45, 0) -> (0.45, -2.82)
  line L25 (0.45, -2.82) -> (-0.45, -2.82)
  line L26 (-0.45, -2.82) -> (-0.45, 0)
  line L27 (1.55, -2.82) -> (1.55, 6.4) projected
  line L28 (1.55, 0) -> (2.95, 0)
  line L29 (2.95, 0) -> (2.95, -2.82)
  line L30 (2.95, -2.82) -> (1.55, -2.82)
  line L31 (1.55, -2.82) -> (1.55, 0)
  line L32 (4.05, -2.82) -> (4.05, 6.4) projected
  line L33 (4.05, 0) -> (6.25, 0)
  line L34 (6.25, 0) -> (6.25, -2.62)
  line L35 (5.2, -2.82) -> (4.05, -2.82)
  line L36 (4.05, -2.82) -> (4.05, 0)
  line L37 (6.55, -5.82) -> (5.2, -5.82)
  line L38 (5.2, -5.82) -> (5.2, -2.82)
  line L39 (6.25, -2.62) -> (6.55, -2.62)
  line L40 (6.55, -2.62) -> (6.55, -5.82)
  line L41 (5.2, -5.82) -> (5.2, -2.82) projected
  line L42 (6.55, -5.82) -> (5.2, -5.82) projected
  line L43 (6.55, -2.62) -> (6.55, -5.82) projected
  line L44 (6.25, -2.62) -> (6.55, -2.62) projected
  line L45 (5.55, 0) -> (6.25, 0) projected
  line L46 (6.25, 0) -> (6.25, -2.62) projected
  line L47 (5.2, -2.82) -> (4.05, -2.82) projected
  point P0 (0, 0)
  constraints: 56 end point, 14 parallel, 12 point on line, 10 collinear, 7 horizontal, 7 perpendicular
extrude "Extrusion12" add sketch "Sketch12" along normal blind 0.68
sketch "Sketch13" plane through (0, -0.68, 0) normal (0, -1, 0) x (1, 0, 0)
  line L0 (-1.55, -2.82) -> (-2.95, -2.82) projected
  line L1 (-2.65, -2.82) -> (-1.85, -2.82)
  line L2 (-1.85, -2.82) -> (-1.85, -0.82)
  line L3 (-2.65, -0.82) -> (-2.65, -2.82)
  line L4 (0.45, -2.82) -> (-0.45, -2.82) projected
  line L5 (-0.15, -2.82) -> (0.15, -2.82)
  line L6 (0.15, -2.82) -> (0.15, -0.82)
  line L7 (-0.15, -0.82) -> (-0.15, -2.82)
  line L8 (2.95, -2.82) -> (1.55, -2.82) projected
  line L9 (1.85, -2.82) -> (2.65, -2.82)
  line L10 (2.65, -2.82) -> (2.65, -0.82)
  line L11 (1.85, -0.82) -> (1.85, -2.82)
  line L12 (2.95, 6.4) -> (2.95, -2.82) projected
  line L13 (1.395, 0) -> (2.605, 0) projected
  line L14 (1.55, -0.82) -> (1.55, 0)
  line L15 (1.55, 0) -> (2.95, 0)
  line L16 (2.95, 0) -> (2.95, -0.82)
  line L17 (0.45, 6.4) -> (0.45, -2.82) projected
  line L18 (-0.45, -2.82) -> (-0.45, 6.4) projected
  line L19 (0.45, 0) -> (-0.45, 0)
  line L20 (-0.45, 0) -> (-0.45, -0.82)
  line L21 (0.45, -0.82) -> (0.45, 0)
  line L22 (-1.55, 6.4) -> (-1.55, -2.82) projected
  line L23 (-2.95, -2.82) -> (-2.95, 6.4) projected
  line L24 (-1.55, 0) -> (-2.95, 0)
  line L25 (-2.95, 0) -> (-2.95, -0.82)
  line L26 (-1.55, -0.82) -> (-1.55, 0)
  line L27 (0, -9.014) -> (0, 13.344) projected
  line L28 (0.75, 6.9) -> (0.75, -4.62) projected
  line L29 (1.55, 0) -> (1.55, -2.82) projected
  line L30 (-2.95, -0.82) -> (-2.65, -0.82)
  line L31 (-1.85, -0.82) -> (-1.55, -0.82)
  line L32 (-0.45, -0.82) -> (-0.15, -0.82)
  line L33 (0.15, -0.82) -> (0.45, -0.82)
  line L34 (2.95, -0.82) -> (2.65, -0.82)
  line L35 (1.85, -0.82) -> (1.55, -0.82)
  line L36 (4.05, 0) -> (4.05, -2.82) projected
  line L37 (4.05, 0) -> (6.25, 0)
  line L38 (4.35, -0.82) -> (4.05, -0.82)
  line L39 (4.05, -0.82) -> (4.05, 0)
  line L40 (6.25, 0) -> (6.25, -5.82)
  line L41 (5.2, -2.82) -> (4.35, -2.82)
  line L42 (4.35, -2.82) -> (4.35, -0.82)
  line L43 (6.25, -5.82) -> (5.2, -5.82) projected
  line L44 (5.2, -5.82) -> (6.25, -5.82)
  line L45 (5.2, -2.82) -> (5.2, -5.82)
  line L46 (4.05, -2.82) -> (5.2, -2.82) projected
  line L47 (5.2, -2.82) -> (5.2, -5.82) projected
  line L48 (-4.05, 0) -> (-6.25, 0) projected
  line L49 (-6.25, 0) -> (-4.4, 0)
  line L50 (-4.05, 6.4) -> (-4.05, -2.82) projected
  line L51 (-6.25, 0) -> (-4.05, 0)
  line L52 (-4.05, 0) -> (-4.05, -0.82)
  line L53 (-4.05, -0.82) -> (-4.35, -0.82)
  line L54 (-5.2, -5.82) -> (-6.25, -5.82) projected
  line L55 (-6.25, 0) -> (-5.2, 0)
  line L56 (-5.2, -2.82) -> (-5.2, -5.82)
  line L57 (-5.2, -5.82) -> (-6.25, -5.82)
  line L58 (-6.25, -5.82) -> (-6.25, 0)
  line L59 (-5.2, -2.82) -> (-4.35, -2.82)
  line L60 (-4.75, 6.9) -> (-4.75, -4.62) projected
  line L61 (-4.35, -2.82) -> (-4.35, -0.82)
  line L62 (-5.2, -2.82) -> (-4.05, -2.82) projected
  point P0 (0, 0)
  point P1 (2.605, 0)
  point P2 (-6.25, -5.82)
  dimension "d289" = 2
  dimension "d293" = 0.3
  dimension "d294" = 0.3
  dimension "d295" = 0.3
  dimension "d296" = 0.3
  dimension "d297" = 0.3
  dimension "d298" = 0.3
  dimension "d299" = 0.3
  constraints: 84 end point, 17 parallel, 12 collinear, 12 horizontal, 12 point on line, 11 perpendicular, 1 other
  measures "d289" distance between parallel lines of L1 L30
  measures "d293" distance between parallel lines of L17 L6
  measures "d294" distance between parallel lines of L23 L3
  measures "d295" distance between parallel lines of L12 L10
  measures "d296" distance between parallel lines of L36 L42
  measures "d297" distance between parallel lines of L22 L2
  measures "d298" distance between parallel lines of L29 L11
  measures "d299" distance between parallel lines of L61 L50
extrude "Extrusion13" add sketch "Sketch13" along normal blind 0.2 contours L0 L3 L30 L23 L24 L22 L31 L2 | L4 L27 L19 L17 L33 L6 | L4 L7 L32 L18 L19 L27 | L8 L11 L35 L14 L13 L15 L12 L34 L10 | L37 L40 L43 L45 L41 L42 L38 L36 | L50 L53 L61 L59 L60 L48 | L60 L59 L56 L54 L58 L48
sketch "Sketch14" plane through (0, -0.88, 0) normal (0, -1, 0) x (1, 0, 0)
  line L0 (-6.25, -4.62) -> (-6.25, 0) projected
  line L1 (-6.25, 0) -> (-4.05, 0)
  line L2 (-4.05, 0) -> (-4.05, -2.82)
  line L3 (-4.05, -2.82) -> (-5.2, -2.82)
  line L4 (-6.25, -2.82) -> (-6.25, 0)
  line L5 (-5.2, -2.82) -> (-4.35, -2.82) projected
  line L6 (-5.2, -2.82) -> (-5.2, -4.32)
  line L7 (-5.2, -4.32) -> (-5.7, -4.32)
  line L8 (-6.25, -4.32) -> (-6.25, -2.82)
  line L9 (-5.2, -5.82) -> (-5.2, -2.82) projected
  line L10 (-5.7, -4.32) -> (-5.7, -5.82)
  line L11 (-5.7, -5.82) -> (-6.25, -5.82)
  line L12 (-6.25, -5.82) -> (-6.25, -4.32)
  line L13 (-6.25, -5.82) -> (-5.2, -5.82) projected
  line L14 (-4.05, -0.82) -> (-4.05, 0) projected
  line L15 (4.05, 0) -> (6.25, 0)
  line L16 (5.2, -2.82) -> (4.05, -2.82)
  line L17 (4.05, -2.82) -> (4.05, 0)
  line L18 (6.25, 0) -> (6.25, -5.82)
  line L19 (5.7, -4.32) -> (5.2, -4.32)
  line L20 (5.2, -4.32) -> (5.2, -2.82)
  line L21 (6.25, -5.82) -> (5.7, -5.82)
  line L22 (5.7, -5.82) -> (5.7, -4.32)
  line L23 (6.25, 0) -> (4.05, 0) projected
  line L24 (4.35, -2.82) -> (5.2, -2.82) projected
  line L25 (4.05, 0) -> (4.05, -0.82) projected
  line L26 (5.2, -2.82) -> (5.2, -5.82) projected
  line L27 (5.2, -5.82) -> (6.25, -5.82) projected
  line L28 (6.25, -5.82) -> (6.25, 0) projected
  line L29 (-2.95, 0) -> (-2.95, -0.82) projected
  line L30 (-2.95, 0) -> (-1.55, 0)
  line L31 (-1.55, 0) -> (-1.55, -2.82)
  line L32 (-1.55, -2.82) -> (-2.95, -2.82)
  line L33 (-2.95, -2.82) -> (-2.95, 0)
  line L34 (-0.45, 0) -> (-0.45, -0.82) projected
  line L35 (0.45, 6.4) -> (0.45, -2.82) projected
  line L36 (-0.45, 0) -> (0.45, 0)
  line L37 (0.45, 0) -> (0.45, -2.82)
  line L38 (0.45, -2.82) -> (-0.45, -2.82)
  line L39 (-0.45, -2.82) -> (-0.45, 0)
  line L40 (1.55, 0) -> (2.95, 0) projected
  line L41 (2.95, -2.82) -> (1.55, -2.82) projected
  line L42 (1.55, 0) -> (2.95, 0)
  line L43 (2.95, 0) -> (2.95, -2.82)
  line L44 (2.95, -2.82) -> (1.55, -2.82)
  line L45 (1.55, -2.82) -> (1.55, 0)
  point P0 (1.55, -2.82)
  point P1 (-0.45, -0.82)
  dimension "d302" = 2.2
  dimension "d304" = 0.55
  dimension "d305" = 1.5
  dimension "d307" = 0.55
  constraints: 61 end point, 12 parallel, 11 collinear, 5 horizontal, 5 perpendicular, 1 point on line
  measures "d302" distance of L2.end L4.start
  measures "d304" distance of L10.end L11.end
  measures "d305" distance between parallel lines of L7 L3
  measures "d307" distance between parallel lines of L18 L22
extrude "Extrusion14" add sketch "Sketch14" along normal blind 0.1 contours L0 L1 L2 L3 L6 L7 L10 L11 L12 | L15 L18 L21 L22 L19 L20 L16 L17 | L30 L31 L32 L33 L29 | L36 L35 L38 L39 L34 | L40 L43 L41 L45
sketch "Sketch15" plane through (-6.25, -0.98, -5.82) normal (0, -1, 0) x (0, 0, 1)
  line L0 (5.82, 0) -> (5.82, -12.5) projected
  line L1 (5.82, -12.5) -> (1.2, -12.5) projected
  line L2 (5.82, 0) -> (3, 0)
  line L3 (3, -1.05) -> (3, -11.45)
  line L4 (3, -12.5) -> (5.82, -12.5)
  line L5 (5.82, -12.5) -> (5.82, 0)
  line L6 (3, -5.8) -> (3, -6.7) projected
  line L7 (1.5, -1.05) -> (3, -1.05) projected
  line L8 (3, 0) -> (0, 0)
  line L9 (1.5, -0.55) -> (1.5, -1.05)
  line L10 (1.5, -1.05) -> (3, -1.05)
  line L11 (1.2, -11.45) -> (3, -11.45) projected
  line L12 (3.2, -12.5) -> (0, -12.5) projected
  line L13 (3, -11.45) -> (1.5, -11.45)
  line L14 (1.5, -11.45) -> (1.5, -11.95)
  line L15 (1.5, -12.5) -> (3, -12.5)
  line L16 (1.5, -11.95) -> (0, -11.95) projected
  line L17 (1.5, -11.95) -> (0, -11.95)
  line L18 (0, -11.95) -> (0, -12.5)
  line L19 (0, -12.5) -> (1.5, -12.5)
  line L20 (1.5, -0.55) -> (0, -0.55)
  line L21 (0, -0.55) -> (0, 0)
  line L22 (0, -0.55) -> (1.5, -0.55) projected
  line L23 (0, 0) -> (0, -0.55) projected
  line L24 (0, -11.95) -> (0, -12.5) projected
  point P0 (5.82, -6.25)
  constraints: 30 end point, 5 horizontal, 5 parallel, 5 perpendicular, 4 collinear, 4 point on line
extrude "Extrusion15" add sketch "Sketch15" along normal blind 0.5
sketch "Sketch16" plane through (-6.25, -1.48, -5.82) normal (0, -1, 0) x (1, 0, 0)
  line L0 (0, 1.2) -> (0, 5.82) projected
  line L1 (12.5, 0) -> (12.5, 3.2) projected
  line L2 (0, 5.82) -> (12.5, 5.82)
  line L3 (12.5, 5.82) -> (12.5, 2.52)
  line L4 (12.5, 2.52) -> (0, 2.52)
  line L5 (0, 2.52) -> (0, 5.82)
  line L6 (1.05, 1.5) -> (0.55, 1.5) projected
  line L7 (0, 2.52) -> (1.05, 2.52)
  line L8 (1.05, 2.52) -> (1.05, 1.5)
  line L9 (1.05, 1.5) -> (0, 1.5)
  line L10 (0, 1.5) -> (0, 2.52)
  line L11 (0, 1.5) -> (0.55, 1.5)
  line L12 (0.55, 1.5) -> (0.55, 0)
  line L13 (0.55, 0) -> (0, 0)
  line L14 (0, 0) -> (0, 1.5)
  line L15 (11.45, 1.2) -> (11.45, 3) projected
  line L16 (12.5, 2.52) -> (11.45, 2.52)
  line L17 (11.45, 2.52) -> (11.45, 1.5)
  line L18 (11.45, 1.5) -> (12.5, 1.5)
  line L19 (12.5, 1.5) -> (12.5, 2.52)
  line L20 (11.95, 0) -> (11.95, 1.5) projected
  line L21 (12.5, 1.5) -> (11.95, 1.5)
  line L22 (11.95, 1.5) -> (11.95, 0)
  line L23 (11.95, 0) -> (12.5, 0)
  line L24 (12.5, 0) -> (12.5, 1.5)
  line L25 (0.55, 0) -> (0.55, 1.5) projected
  line L26 (0, 0) -> (0.55, 0) projected
  point P0 (6.25, 5.82)
  dimension "d312" = 3.3
  constraints: 40 end point, 10 parallel, 5 horizontal, 5 perpendicular, 3 point on line, 2 collinear
  measures "d312" distance of L2.end L3.end
extrude "Extrusion16" add sketch "Sketch16" along normal blind 0.4
sketch "Sketch17" plane through (-6.25, -1.88, -5.82) normal (0, -1, 0) x (1, 0, 0)
  line L0 (12.5, 5.82) -> (0, 5.82) projected
  line L1 (12.5, 3.2) -> (12.5, 0) projected
  line L2 (0, 5.82) -> (12.5, 5.82)
  line L3 (12.5, 5.82) -> (12.5, 2.52)
  line L4 (12.5, 2.52) -> (0, 2.52)
  line L5 (0, 2.52) -> (0, 5.82)
  line L6 (1.05, 2.52) -> (11.45, 2.52) projected
  line L7 (1.05, 0) -> (1.05, 1.5) projected
  line L8 (0, 2.52) -> (1.05, 2.52)
  line L9 (1.05, 2.52) -> (1.05, 0)
  line L10 (1.05, 0) -> (0, 0)
  line L11 (0, 0) -> (0, 2.52)
  line L12 (11.45, 1.5) -> (11.45, 0) projected
  line L13 (12.5, 2.52) -> (11.45, 2.52)
  line L14 (11.45, 2.52) -> (11.45, 0)
  line L15 (11.45, 0) -> (12.5, 0)
  line L16 (12.5, 0) -> (12.5, 2.52)
  point P0 (6.25, 5.82)
  constraints: 24 end point, 6 parallel, 3 horizontal, 3 perpendicular, 1 collinear, 1 point on line
extrude "Extrusion17" add sketch "Sketch17" along normal blind 0.98
sketch "Sketch18" plane through (-6.25, -2.86, -5.82) normal (0, -1, 0) x (1, 0, 0)
  line L0 (1.05, 1.2) -> (1.05, 0) projected
  line L1 (1.05, 0) -> (11.45, 0)
  line L2 (11.45, 0) -> (11.45, 3)
  line L3 (11.45, 3) -> (1.05, 3)
  line L4 (1.05, 3) -> (1.05, 0)
  line L5 (11.45, 2.52) -> (11.45, 0) projected
  point P0 (6.25, 5.82)
  dimension "d317" = 3
  constraints: 8 end point, 2 parallel, 1 collinear, 1 horizontal, 1 perpendicular
  measures "d317" distance of L2.end L1.end
extrude "Extrusion18" cut sketch "Sketch18" against normal blind 0.68
sketch "Sketch20" plane through (-6.25, -2.86, -5.82) normal (0, -1, 0) x (1, 0, 0)
  line L0 (2, 3) -> (2, 10.7)
  line L1 (2, 10.7) -> (0, 10.7)
  line L2 (10.5, 3) -> (10.5, 10.7)
  line L3 (10.5, 10.7) -> (12.5, 10.7)
  line L4 (0, 0) -> (1.05, 0) projected
  line L5 (12.5, 0) -> (12.5, 3.2) projected
  line L6 (12.5, 0) -> (11.45, 0)
  line L7 (11.45, 0) -> (11.45, 3)
  line L8 (12.5, 10.7) -> (12.5, 0)
  line L9 (1.05, 0) -> (1.05, 1.5) projected
  line L10 (1.05, 0) -> (0, 0)
  line L11 (0, 0) -> (0, 10.7)
  line L12 (1.05, 3) -> (1.05, 0)
  line L13 (11.45, 3) -> (11.45, 0) projected
  line L14 (1.05, 3) -> (2, 3)
  line L15 (1.05, 3) -> (11.45, 3) projected
  line L16 (0, 5.82) -> (0, 0) projected
  line L17 (11.45, 3) -> (10.5, 3)
  point P0 (0, 0)
  dimension "d327" = 2
  dimension "d328" = 10.7
  constraints: 24 end point, 6 perpendicular, 5 collinear, 2 horizontal, 2 parallel, 1 point on line
  measures "d327" distance of L2.end L3.end
  measures "d328" distance between parallel lines of L1 L4
extrude "Extrusion20" add sketch "Sketch20" along normal blind 1.15
sketch "Sketch21" plane through (-6.25, 0.32, -5.82) normal (-1, 0, 0) x (0, 0, 1)
  line L0 (5.82, -3.18) -> (3, -3.18) projected
  line L1 (3, -3.18) -> (5.82, -3.18) projected
  line L2 (5.82, -3.18) -> (3, -3.18) projected
  line L3 (5.82, -3.18) -> (10.7, -3.18) projected
  line L4 (10.7, -3.18) -> (10.7, -4.33) projected
  line L5 (3, -4.33) -> (10.7, -4.33) projected
  line L6 (3, -3.18) -> (3, -4.33) projected
  line L7 (5.82, -0.32) -> (5.82, -1.3) projected
  line L8 (5.82, -0.32) -> (5.82, 1.52) projected
  line L9 (5.82, 1.52) -> (5.82, 1.74) projected
  line L10 (5.82, 1.52) -> (5.82, 1.74) projected
  line L11 (5.82, 1.52) -> (5.82, 1.74) projected
  line L12 (5.82, 1.52) -> (5.82, 1.74) projected
  line L13 (5.82, 1.52) -> (5.82, 1.74) projected
  line L14 (5.82, 1.52) -> (5.82, 1.74) projected
  line L15 (5.82, 1.52) -> (5.82, 1.74) projected
  line L16 (5.82, 1.52) -> (5.82, 1.74) projected
  line L17 (5.82, 1.52) -> (5.82, 1.74) projected
  line L18 (5.82, 1.52) -> (5.82, 1.74) projected
  line L19 (5.82, -0.32) -> (5.82, 1.52) projected
  line L20 (5.82, -0.32) -> (5.82, -1.3) projected
  line L21 (5.82, -0.32) -> (5.82, -1.3) projected
  line L22 (5.82, -0.32) -> (5.82, -1.3) projected
  line L23 (5.82, -0.32) -> (5.82, -1.3) projected
  line L24 (5.82, -0.32) -> (5.82, -1.3) projected
  line L25 (5.82, -0.32) -> (5.82, -1.3) projected
  line L26 (5.82, -0.32) -> (5.82, -1.3) projected
  line L27 (5.82, -3.18) -> (5.82, 2.24) projected
  line L28 (5.82, -3.18) -> (5.82, 2.24) projected
  line L29 (5.82, -3.18) -> (5.82, 2.24) projected
  line L30 (3, -3.18) -> (5.82, -3.18)
  line L31 (5.82, -3.18) -> (3, -3.5)
  line L32 (3, -4.33) -> (3, -2.5) projected
  line L33 (3, -3.18) -> (3, -3.5)
  dimension "d332" = 0.32
  constraints: 6 end point, 1 collinear, 1 perpendicular, 1 point on line, 1 other
  measures "d332" distance of L31.end L0.end
extrude "Extrusion21" add sketch "Sketch21" against normal up to surface (12.5 mm away) contours L31 L6 L0
ref_plane "Work Plane1" through (-6.25, -3.18, -2.82) normal (0, -1, 0) x (1, 0, 0)
sketch "Sketch19" plane through (-6.25, -3.18, -5.82) normal (0, -1, 0) x (1, 0, 0)
  line L0 (5.5, 5.88) -> (7, 5.88)
  line L1 (7, 5.88) -> (7, 3.88)
  line L2 (7, 3.88) -> (5.5, 3.88)
  line L3 (5.5, 3.88) -> (5.5, 5.88)
  line L4 (12.5, 5.82) -> (0, 5.82) projected
  line L5 (10.5, 3) -> (11.45, 3) projected
  line L6 (11.45, 3) -> (11.45, 0) projected
  line L7 (11.45, 0) -> (12.5, 0) projected
  line L8 (12.5, 0) -> (12.5, 10.7) projected
  line L9 (12.5, 10.7) -> (10.5, 10.7) projected
  line L10 (10.5, 10.7) -> (10.5, 3) projected
  point P0 (6.25, 5.82)
  dimension "d320" = 1.5
  dimension "d321" = 2
  dimension "d322" = 0.06
  dimension "d336" = 5.5
  constraints: 8 end point, 2 parallel, 1 horizontal, 1 perpendicular
  measures "d320" distance of L1.end L2.end
  measures "d321" distance of L2.end L0.start
  measures "d322" distance between parallel lines of L0 L4
  measures "d336" distance between parallel lines of L1 L8
extrude "Extrusion19" cut sketch "Sketch19" against normal blind 0.62 contours L0 L1 L4 L3 | L4 L1 L2 L3